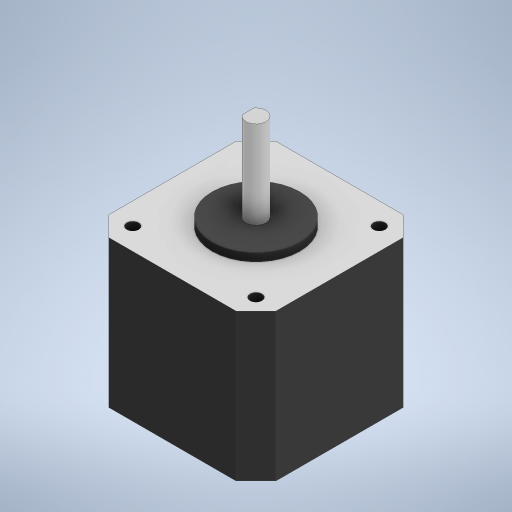
# Autodesk Inventor part: 스텝모터 4401
Saved by Autodesk Inventor 2023 (Build 270158000, 158)
## iProperties
Created: 2022-11-10
Part Number: 스텝모터 4401
Material: 일반
Document SubType Name: Modeling
Designer: user
Density: 1 g/cm^3
Appearance: 기본값
Author: user
Autodesk Inventor part; units mm, degrees
ref_plane "YZ Plane" through (0, 0, 0) normal (1, 0, 0) x (0, 1, 0)
ref_plane "XZ Plane" through (0, 0, 0) normal (0, 1, 0) x (-1, 0, 0)
ref_plane "XY Plane" through (0, 0, 0) normal (0, 0, 1) x (1, 0, 0)
sketch "스케치1" plane through (0, 0, 0) normal (0, 1, 0) x (-1, 0, 0)
  line L0 (-16, 21) -> (16, 21)
  line L1 (21, 16) -> (21, -16)
  line L2 (16, -21) -> (-16, -21)
  line L3 (-21, -16) -> (-21, 16)
  line L4 (-21, 21) -> (21, -21) construction
  line L5 (21, 21) -> (-21, -21) construction
  line L6 (16, 21) -> (21, 16)
  line L7 (21, -16) -> (16, -21)
  line L8 (-16, -21) -> (-21, -16)
  line L9 (-21, 16) -> (-16, 21)
  point P0 (0, 0)
  dimension "d0" = 42
  dimension "d1" = 42
  dimension "d2" = 5
  dimension "d3" = 5
  dimension "d4" = 5
  dimension "d5" = 5
  dimension "d6" = 5
  dimension "d7" = 5
  dimension "d8" = 5
  dimension "d9" = 5
  constraints: 20 end point, 8 point on line, 2 midpoint, 2 parallel, 1 horizontal, 1 perpendicular
  measures "d0" distance of L4.end L5.end
  measures "d1" distance of L5.start L4.end
  measures "d2" distance of L0.end L5.start
  measures "d3" distance of L1.start L5.start
  measures "d4" distance of L1.end L4.end
  measures "d5" distance of L2.start L4.end
  measures "d6" distance of L2.end L5.end
  measures "d7" distance of L3.start L5.end
  measures "d8" distance of L3.end L4.start
  measures "d9" distance of L0.start L4.start
extrude "돌출1" add sketch "스케치1" against normal blind 37
sketch "스케치2" plane through (0, 0, 0) normal (0, 1, 0) x (1, 0, 0)
  circle A0 centre (-15.5, -15.5) radius 1.5
  line L0 (0, 0) -> (-5.5004, 0) construction
  line L1 (0, 0) -> (0, 5.7427) construction
  circle A1 centre (-15.5, 15.5) radius 1.5
  circle A2 centre (15.5, -15.5) radius 1.5
  circle A3 centre (15.5, 15.5) radius 1.5
  dimension "d12" = 3
  dimension "d13" = 31
  dimension "d14" = 31
  constraints: 4 centre point, 4 end point, 3 symmetric about line, 1 horizontal, 1 vertical, 3 other
  measures "d12" diameter of A0
  measures "d13" distance of A3.centre A1.centre
  measures "d14" distance of A2.centre A3.centre
extrude "돌출2" cut sketch "스케치2" against normal blind 10
sketch "스케치3" plane through (0, 0, 0) normal (0, 1, 0) x (1, 0, 0)
  circle A0 centre (0, 0) radius 11
  dimension "d17" = 22
  constraints: 1 centre point, 1 coincident
  measures "d17" diameter of A0
extrude "돌출3" add sketch "스케치3" along normal blind 2
sketch "스케치4" plane through (0, 2, 0) normal (0, 1, 0) x (1, 0, 0)
  circle A0 centre (0, 0) radius 2.5
  line L0 (-2, -3.7589) -> (-2, 6.4181)
  point P0 (-2, 1.5)
  point P1 (-2, -1.5)
  dimension "d20" = 5
  dimension "d23" = 2
  constraints: 2 end point, 1 centre point, 1 coincident, 1 vertical
  measures "d20" diameter of A0
  measures "d23" distance from line of L0 point (0, 0)
extrude "돌출4" add sketch "스케치4" along normal blind 22 contours A0 L0 picked at (-0.5259, 0.206)
equation "\"d3\" = d2"
equation "\"d4\" = d2"
equation "\"d5\" = d4"
equation "\"d6\" = d2"
equation "\"d7\" = d6"
equation "\"d8\" = d2"
equation "\"d9\" = d8"
